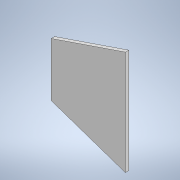
# Autodesk Inventor part: weight
Saved by Autodesk Inventor 2022 (Build 260153000, 153)
## iProperties
Created: 2022-04-15
Part Number: weight
Material: Generic
Document SubType Name: Modeling
Designer: Martijn
Density: 1 g/cm^3
Appearance: Default
Author: Martijn
Autodesk Inventor part; units mm, degrees
ref_plane "YZ Plane" through (0, 0, 0) normal (1, 0, 0) x (0, 1, 0)
ref_plane "XZ Plane" through (0, 0, 0) normal (0, 1, 0) x (-1, 0, 0)
ref_plane "XY Plane" through (0, 0, 0) normal (0, 0, 1) x (1, 0, 0)
sketch "Sketch1" plane through (0, 0, 0) normal (0, 0, 1) x (1, 0, 0)
  line L0 (0, 80) -> (0, -80)
  line L1 (0, -80) -> (220, -155)
  line L2 (220, -155) -> (220, 155)
  line L3 (220, 155) -> (0, 80)
  point P0 (0, 0)
  point P1 (0, 0)
  dimension "d0" = 160
  dimension "d1" = 310
  dimension "d2" = 220
  constraints: 8 end point, 1 coincident, 1 equal length, 1 midpoint, 1 parallel, 1 vertical
  measures "d0" distance of L0.start L0.end
  measures "d1" distance of L1.end L2.end
  measures "d2" distance between parallel lines of L0 L2
extrude "Extrusion1" add sketch "Sketch1" along normal blind 10
body "Solid1"
